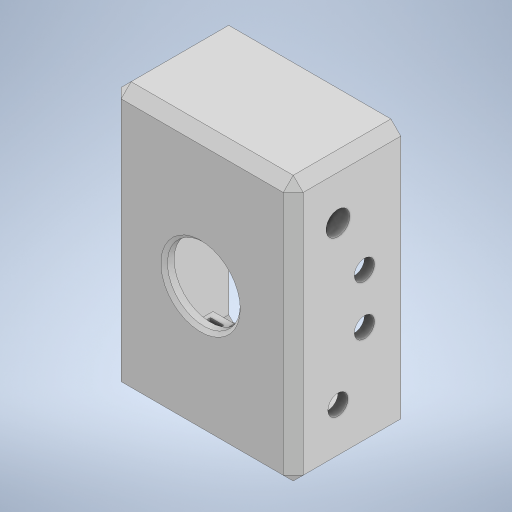
# Autodesk Inventor part: Nixie Tester TOP
Saved by Autodesk Inventor 2024 (Build 280153000, 153)
## iProperties
Created: 2025-09-18
Part Number: Nixie Tester TOP
Material: Generic
Document SubType Name: Modeling
Designer: Login
Density: 1 g/cm^3
Appearance: Default
Author: Login
Autodesk Inventor part; units mm, degrees
ref_plane "YZ Plane" through (0, 0, 0) normal (1, 0, 0) x (0, 1, 0)
ref_plane "XZ Plane" through (0, 0, 0) normal (0, 1, 0) x (-1, 0, 0)
ref_plane "XY Plane" through (0, 0, 0) normal (0, 0, 1) x (1, 0, 0)
sketch "Sketch2" plane through (0, 0, 0) normal (0, 0, 1) x (1, 0, 0)
  line L0 (-27.5, 40) -> (27.5, 40)
  line L1 (27.5, 40) -> (27.5, -40)
  line L2 (27.5, -40) -> (-27.5, -40)
  line L3 (-27.5, -40) -> (-27.5, 40)
  line L4 (-27.5, 40) -> (27.5, -40) construction
  line L5 (27.5, 40) -> (-27.5, -40) construction
  point P0 (0, 0)
  dimension "d4" = 55
  dimension "d5" = 80
  constraints: 12 end point, 2 midpoint, 2 parallel, 1 horizontal, 1 perpendicular
  measures "d4" distance of L1.end L2.end
  measures "d5" distance of L0.end L1.end
extrude "Extrusion2" add sketch "Sketch2" along normal blind 32.5
chamfer "Chamfer1" distance 3 angle 45 8 edges at (27.5, -40, 16.25) (27.5, 40, 16.25) (27.5, 0, 32.5) (0, 40, 32.5) (-27.5, 0, 32.5) (-27.5, -40, 16.25) (0, -40, 32.5) (-27.5, 40, 16.25)
shell "Shell1" thickness 3 removed faces 1 at (-9.1667, 12.3333, 0)
sketch "Sketch3" plane through (23.2574, 35.7574, 29.5) normal (0, 0, -1) x (-1, 0, 0)
  line L0 (45.0074, -1.5074) -> (38.5074, -1.5074)
  line L1 (38.5074, -1.5074) -> (38.5074, -8.0074)
  line L2 (38.5074, -8.0074) -> (45.0074, -8.0074)
  line L3 (45.0074, -8.0074) -> (45.0074, -1.5074)
  line L4 (45.0074, -1.5074) -> (38.5074, -8.0074) construction
  line L5 (38.5074, -1.5074) -> (45.0074, -8.0074) construction
  line L6 (47.7574, 0) -> (47.7574, -71.5147) projected
  line L7 (-1.2426, 4.2426) -> (47.7574, 4.2426) projected
  line L8 (43.7574, -5.9121) -> (41.7574, -7.0668)
  line L9 (41.7574, -7.0668) -> (39.7574, -5.9121)
  line L10 (39.7574, -5.9121) -> (39.7574, -3.6027)
  line L11 (39.7574, -3.6027) -> (41.7574, -2.448)
  line L12 (41.7574, -2.448) -> (43.7574, -3.6027)
  line L13 (43.7574, -3.6027) -> (43.7574, -5.9121)
  line L14 (39.7574, -5.9121) -> (39.7574, -8.0074)
  line L15 (43.7574, -5.9121) -> (43.7574, -8.0074)
  point P0 (23.2574, -35.7574)
  point P1 (41.7574, -4.7574)
  point P2 (41.7574, -4.7574)
  point P3 (43.7574, -4.7574)
  point P4 (39.7574, -4.7574)
  dimension "d12" = 6.5
  dimension "d13" = 6.5
  dimension "d14" = 6
  dimension "d15" = 9
  dimension "d16" = 4
  constraints: 28 end point, 4 midpoint, 3 parallel, 3 perpendicular, 2 point on line, 1 coincident, 1 horizontal, 13 other
  measures "d12" distance of L2.end L1.end
  measures "d13" distance of L1.end L0.end
  measures "d14" distance from line of point (41.757, -4.757) L6
  measures "d15" distance from line of L7 point (41.757, -4.757)
  measures "d16" distance of point (43.757, -4.757) point (39.757, -4.757)
extrude "Extrusion3" add sketch "Sketch3" along normal blind 2 contours L3 L2 L15 L13 L12 L11 L10 L14 L1 L0
sketch "Sketch4" plane through (23.2574, 35.7574, 27.5) normal (0, 0, -1) x (-1, 0, 0)
  line L0 (38.5074, -1.5074) -> (45.0074, -1.5074)
  line L1 (45.0074, -1.5074) -> (45.0074, -8.0074)
  line L2 (45.0074, -8.0074) -> (38.5074, -8.0074)
  line L3 (38.5074, -8.0074) -> (38.5074, -1.5074)
  line L4 (38.5074, -1.5074) -> (45.0074, -8.0074) construction
  line L5 (45.0074, -1.5074) -> (38.5074, -8.0074) construction
  line L6 (38.5074, -1.5074) -> (38.5074, -8.0074) projected
  line L7 (43.7574, -8.0074) -> (45.0074, -8.0074) projected
  circle A0 centre (41.7574, -4.7574) radius 1.05
  point P0 (23.2574, -35.7574)
  dimension "d19" = 6.5
  dimension "d20" = 6.5
  dimension "d21" = 2.1
  constraints: 12 end point, 2 collinear, 2 midpoint, 2 parallel, 1 centre point, 1 coincident, 1 horizontal, 1 perpendicular
  measures "d19" distance of L1.end L2.end
  measures "d20" distance of L0.end L1.end
  measures "d21" diameter of A0
extrude "Extrusion4" add sketch "Sketch4" along normal blind 2
mirror "Mirror1" about plane through (0, 0, 0) normal (0, 1, 0) of "Extrusion4", "Extrusion3"
sketch "Sketch5" plane through (23.2574, 35.7574, 29.5) normal (0, 0, -1) x (-1, 0, 0)
  line L0 (20.5074, -17.5074) -> (27.0074, -17.5074)
  line L1 (27.0074, -17.5074) -> (27.0074, -24.0074)
  line L2 (27.0074, -24.0074) -> (20.5074, -24.0074)
  line L3 (20.5074, -24.0074) -> (20.5074, -17.5074)
  line L4 (20.5074, -17.5074) -> (27.0074, -24.0074) construction
  line L5 (27.0074, -17.5074) -> (20.5074, -24.0074) construction
  line L6 (-1.2426, 4.2426) -> (47.7574, 4.2426) projected
  line L7 (50.7574, 1.2426) -> (50.7574, -72.7574) projected
  line L8 (23.7574, -23.0668) -> (21.7574, -21.9121)
  line L9 (21.7574, -21.9121) -> (21.7574, -19.6027)
  line L10 (21.7574, -19.6027) -> (23.7574, -18.448)
  line L11 (23.7574, -18.448) -> (25.7574, -19.6027)
  line L12 (25.7574, -19.6027) -> (25.7574, -21.9121)
  line L13 (25.7574, -21.9121) -> (23.7574, -23.0668)
  line L14 (21.7574, -21.9121) -> (21.7574, -24.0074)
  line L15 (25.7574, -21.9121) -> (25.7574, -24.0074)
  point P0 (23.2574, -35.7574)
  point P1 (23.7574, -20.7574)
  point P2 (23.7574, -20.7574)
  dimension "d24" = 6.5
  dimension "d25" = 6.5
  dimension "d26" = 25
  dimension "d27" = 27
  dimension "d28" = 4
  constraints: 28 end point, 3 parallel, 3 perpendicular, 2 midpoint, 2 point on line, 1 coincident, 1 horizontal, 13 other
  measures "d24" distance of L1.end L2.end
  measures "d25" distance of L0.end L1.end
  measures "d26" distance from line of L6 point (23.757, -20.757)
  measures "d27" distance from line of L7 point (23.757, -20.757)
  measures "d28" distance between parallel lines of L12 L9
extrude "Extrusion5" add sketch "Sketch5" along normal blind 2 contours L0 L1 L2 L15 L12 L11 L10 L9 L14 L3
sketch "Sketch6" plane through (23.2574, 35.7574, 27.5) normal (0, 0, -1) x (-1, 0, 0)
  line L0 (20.5074, -17.5074) -> (27.0074, -17.5074)
  line L1 (27.0074, -17.5074) -> (27.0074, -24.0074)
  line L2 (27.0074, -24.0074) -> (20.5074, -24.0074)
  line L3 (20.5074, -24.0074) -> (20.5074, -17.5074)
  line L4 (20.5074, -17.5074) -> (27.0074, -24.0074) construction
  line L5 (27.0074, -17.5074) -> (20.5074, -24.0074) construction
  line L6 (27.0074, -17.5074) -> (20.5074, -17.5074) projected
  line L7 (27.0074, -24.0074) -> (27.0074, -17.5074) projected
  circle A0 centre (23.7574, -20.7574) radius 1.05
  point P0 (23.2574, -35.7574)
  dimension "d31" = 6.5
  dimension "d32" = 6.5
  dimension "d33" = 2.1
  constraints: 12 end point, 2 collinear, 2 midpoint, 2 parallel, 1 centre point, 1 coincident, 1 horizontal, 1 perpendicular
  measures "d31" distance of L1.end L2.end
  measures "d32" distance of L0.end L1.end
  measures "d33" diameter of A0
extrude "Extrusion6" add sketch "Sketch6" along normal blind 2
mirror "Mirror2" about plane through (0, 0, 0) normal (0, 1, 0) of "Extrusion6", "Extrusion5"
sketch "Sketch7" plane through (23.2574, 35.7574, 29.5) normal (0, 0, -1) x (-1, 0, 0)
  circle A0 centre (41.7574, -4.7574) radius 1.05 projected
  circle A1 centre (41.7574, -4.7574) radius 1.05
  circle A2 centre (23.7574, -20.7574) radius 1.05 projected
  circle A3 centre (23.7574, -20.7574) radius 1.05
  circle A4 centre (23.7574, -50.7574) radius 1.05 projected
  circle A5 centre (23.7574, -50.7574) radius 1.05
  circle A6 centre (41.7574, -66.7574) radius 1.05 projected
  circle A7 centre (41.7574, -66.7574) radius 1.05
  point P0 (23.2574, -35.7574)
  constraints: 4 centre point, 4 coincident
extrude "Extrusion7" cut sketch "Sketch7" against normal blind 2
sketch "Sketch8" plane through (0, 0, 32.5) normal (0, 0, 1) x (1, 0, 0)
  circle A0 centre (-0.5, 0) radius 11
  line L0 (-27.5, 37) -> (-27.5, -37) projected
  line L1 (24.5, 40) -> (-24.5, 40) projected
  point P0 (0, 0)
  dimension "d38" = 27
  dimension "d39" = 40
  dimension "d40" = 22
  constraints: 1 centre point
  measures "d38" distance from line of L0 A0.centre
  measures "d39" distance from line of L1 A0.centre
  measures "d40" diameter of A0
extrude "Extrusion8" cut sketch "Sketch8" against normal through all
chamfer "Chamfer2" distance 1 angle 45 1 edges at (-11.5, 0, 32.5)
sketch "Sketch9" plane through (-27.5, -37, 0) normal (-1, 0, 0) x (0, 0, 1)
  line L0 (24.01, 41.6) -> (12.81, 41.6)
  line L1 (12.81, 41.6) -> (12.81, 32.4)
  line L2 (12.81, 32.4) -> (24.01, 32.4)
  line L3 (24.01, 32.4) -> (24.01, 41.6)
  line L4 (0, 74) -> (0, 0) projected
  line L5 (32.5, 0) -> (32.5, 74) projected
  point P0 (0, 37)
  point P1 (0, 37)
  dimension "d46" = 11.2
  dimension "d47" = 9.2
  dimension "d50" = 4.6
  dimension "d75" = 8.49
  constraints: 8 end point, 2 parallel, 1 horizontal, 1 midpoint, 1 perpendicular
  measures "d46" distance of L2.end L1.end
  measures "d47" distance of L1.end L0.end
  measures "d50" distance from line of L2 point (0, 37)
  measures "d75" distance between parallel lines of L5 L3
extrude "Extrusion9" cut sketch "Sketch9" against normal up to surface (3 mm away)
sketch "Sketch10" plane through (27.5, -37, 0) normal (1, 0, 0) x (0, 0, -1)
  circle A0 centre (-11, 29.5) radius 3.05
  circle A1 centre (-11, 44.5) radius 3.05
  line L0 (-11, 29.5) -> (-11, 44.5) construction
  line L1 (0, 0) -> (0, 74) projected
  point P0 (0, 37)
  point P1 (0, 37)
  dimension "d52" = 6.1
  dimension "d53" = 6.1
  dimension "d54" = 11
  dimension "d55" = 15
  dimension "d56" = 7.5
  constraints: 2 centre point, 2 end point, 1 midpoint, 1 parallel, 1 vertical
  measures "d52" diameter of A0
  measures "d53" diameter of A1
  measures "d54" distance between parallel lines of L1 L0
  measures "d55" distance of L0.start L0.end
  measures "d56" vertical distance of point (0, 37) L0.start
extrude "Extrusion10" cut sketch "Sketch10" against normal up to surface (3 mm away)
sketch "Sketch11" plane through (27.5, -37, 0) normal (1, 0, 0) x (0, 0, -1)
  circle A0 centre (-19, 13.25) radius 3.05
  line L0 (-29.5, -3) -> (0, -3) projected
  line L1 (0, 0) -> (0, 74) projected
  line L2 (-32.5, 74) -> (-32.5, 0) projected
  point P0 (0, 37)
  dimension "d59" = 6.1
  dimension "d60" = 16.25
  dimension "d76" = 13.5
  constraints: 1 centre point
  measures "d59" diameter of A0
  measures "d60" distance from line of L0 A0.centre
  measures "d76" distance from line of A0.centre L2
extrude "Extrusion11" cut sketch "Sketch11" against normal up to surface (3 mm away)
sketch "Sketch12" plane through (27.5, -37, 0) normal (1, 0, 0) x (0, 0, -1)
  circle A0 centre (-19, 60.75) radius 3.6
  circle A1 centre (-19, 13.25) radius 3.05 projected
  line L0 (-19, 13.25) -> (-19, 60.75) construction
  line L1 (0, 77) -> (-29.5, 77) projected
  point P0 (0, 37)
  dimension "d64" = 7.2
  dimension "d65" = 16.25
  constraints: 2 end point, 1 centre point, 1 vertical
  measures "d64" diameter of A0
  measures "d65" distance from line of L1 L0.end
extrude "Extrusion12" cut sketch "Sketch12" against normal up to surface (3 mm away) contours A0
sketch "Sketch14" plane through (24.5, -35.7574, 0) normal (-1, 0, 0) x (0, 0, 1)
  line L0 (12.5, 51.5074) -> (25.5, 51.5074)
  line L1 (25.5, 51.5074) -> (25.5, 67.5074)
  line L2 (25.5, 67.5074) -> (12.5, 67.5074)
  line L3 (12.5, 67.5074) -> (12.5, 51.5074)
  circle A0 centre (19, 59.5074) radius 3.6 projected
  line L4 (12.5, 51.5074) -> (25.5, 67.5074) construction
  line L5 (25.5, 51.5074) -> (12.5, 67.5074) construction
  point P0 (0, 35.7574)
  dimension "d77" = 13
  dimension "d78" = 16
  constraints: 12 end point, 2 midpoint, 2 parallel, 1 horizontal, 1 perpendicular
  measures "d77" distance of L2.end L1.end
  measures "d78" distance of L1.end L0.end
extrude "Extrusion14" add sketch "Sketch14" along normal blind 2.5
sketch "Sketch15" plane through (22, -35.7574, 0) normal (-1, 0, 0) x (0, 0, 1)
  line L0 (17.25, 50.4574) -> (20.75, 50.4574)
  line L1 (20.75, 50.4574) -> (20.75, 52.9574)
  line L2 (20.75, 52.9574) -> (17.25, 52.9574)
  line L3 (17.25, 52.9574) -> (17.25, 50.4574)
  line L4 (17.25, 50.4574) -> (20.75, 52.9574) construction
  line L5 (20.75, 50.4574) -> (17.25, 52.9574) construction
  circle A0 centre (19, 59.5074) radius 3.6 projected
  point P0 (0, 35.7574)
  point P1 (19, 51.7074)
  dimension "d81" = 3.5
  dimension "d82" = 2.5
  dimension "d83" = 7.8
  dimension "d84" = 0
  constraints: 12 end point, 2 midpoint, 2 parallel, 1 horizontal, 1 perpendicular
  measures "d81" distance of L2.end L1.end
  measures "d82" distance of L1.end L0.end
  measures "d83" distance of A0.centre point (19, 51.707)
  measures "d84" horizontal distance of A0.centre point (19, 51.707)
extrude "Extrusion15" cut sketch "Sketch15" against normal up to surface (2.5 mm away) contours L3 L2 L1 L0
fillet "Fillet2" radius 0.5 8 edges at (23.25, 17.2, 20.75) (23.25, 17.2, 17.25) (23.25, 15.75, 17.25) (23.25, 15.75, 20.75) (23.25, 15.75, 12.5) (23.25, 31.75, 12.5) (23.25, 31.75, 25.5) (23.25, 15.75, 25.5)
equation "\"d56\" = 0.5 * d55"
body "Solid2"
